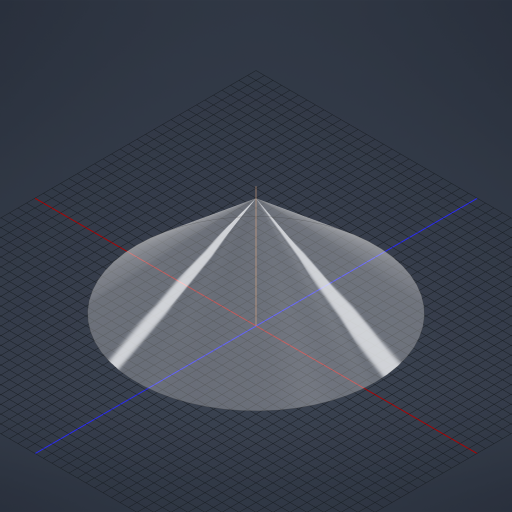
# Autodesk Inventor part: Viewcone
Saved by Autodesk Inventor 2023.2 (Build 272271030, 271C)
## iProperties
Created: 2023-02-20
Part Number: Viewcone
Material: Generisch
Document SubType Name: Modeling
Designer: Stefan
Mass: 154417 g
Surface Area: 22723 cm^2
Volume: 154417 cm^3
Density: 1 g/cm^3
Appearance: Polycarbonat - klar
Author: Stefan
Autodesk Inventor part; units mm, degrees
ref_plane "YZ Plane" through (0, 0, 0) normal (1, 0, 0) x (0, 1, 0)
ref_plane "XZ Plane" through (0, 0, 0) normal (0, 1, 0) x (-1, 0, 0)
ref_plane "XY Plane" through (0, 0, 0) normal (0, 0, 1) x (1, 0, 0)
sketch "Skizze6" plane through (0, 0, 0) normal (0, 0, 1) x (1, 0, 0)
  line L0 (0, 470) -> (-560.1242, 0)
  line L1 (0, 0) -> (-560.1242, 0)
  line L2 (0, 470) -> (0, 0)
  line L3 (0, -94) -> (0, 564) construction
  dimension "d3" = 50
  dimension "d6" = 470
  constraints: 6 end point, 1 collinear, 1 perpendicular
  measures "d3" angle of L0 L2
  measures "d6" distance of L0.start L1.start
revolve "Umdrehung1" add sketch "Skizze6" angle 360 about axis through (0, -10, 0) along (0, 1, 0)
